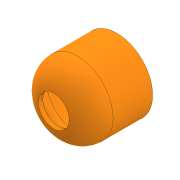
# Autodesk Inventor part: Axis 6 Gearbox
Saved by Autodesk Inventor 2020 (Build 240168000, 168)
## iProperties
Created: 2021-06-29
Part Number: Axis 6 Gearbox
Material: Generic
Document SubType Name: Modeling
Designer: Coy
Density: 1 g/cm^3
Appearance: Orange
Author: Coy
Autodesk Inventor part; units mm, degrees
ref_plane "YZ Plane" through (0, 0, 0) normal (1, 0, 0) x (0, 1, 0)
ref_plane "XZ Plane" through (0, 0, 0) normal (0, 1, 0) x (-1, 0, 0)
ref_plane "XY Plane" through (0, 0, 0) normal (0, 0, 1) x (1, 0, 0)
sketch "Sketch1" plane through (0, 0, 0) normal (0, 0, 1) x (1, 0, 0)
  circle A0 centre (0, 0) radius 6
  dimension "d0" = 12
  constraints: 1 centre point, 1 coincident
  measures "d0" diameter of A0
extrude "Extrusion1" add sketch "Sketch1" against normal blind 8
chamfer "Chamfer1" distance 8 angle 2 1 edges at (-6, 0, -8) measured on face at (-6, 0, -7.5)
sketch "Sketch2" plane through (0, 0, -8) normal (0, 0, -1) x (-1, 0, 0)
  circle A0 centre (0, 0) radius 6 construction
  circle A1 centre (0, 0) radius 5.7206 projected
  line L0 (0, 0) -> (0, 8.298) construction
  arc A2 (0.1999, 5.9933) -> (-0.1999, 5.9933) centre (0, 6) ccw
  line L1 (0.1907, 5.7175) -> (0.2, 5.9967)
  line L2 (-0.1907, 5.7175) -> (-0.2, 5.9967)
  arc A3 (-5.0904, 3.1698) -> (-5.2903, 2.8236) centre (-5.1962, 3) ccw
  line L3 (-5.0468, 2.6936) -> (-5.2933, 2.8251)
  line L4 (-4.8561, 3.0239) -> (-5.0933, 3.1715)
  arc A4 (-5.2903, -2.8236) -> (-5.0904, -3.1698) centre (-5.1962, -3) ccw
  line L5 (-4.8561, -3.0239) -> (-5.0933, -3.1715)
  line L6 (-5.0468, -2.6936) -> (-5.2933, -2.8251)
  arc A5 (-0.1999, -5.9933) -> (0.1999, -5.9933) centre (0, -6) ccw
  line L7 (0.1907, -5.7175) -> (0.2, -5.9967)
  line L8 (-0.1907, -5.7175) -> (-0.2, -5.9967)
  arc A6 (5.0904, -3.1698) -> (5.2903, -2.8236) centre (5.1962, -3) ccw
  line L9 (5.0468, -2.6936) -> (5.2933, -2.8251)
  line L10 (4.8561, -3.0239) -> (5.0933, -3.1715)
  arc A7 (5.2903, 2.8236) -> (5.0904, 3.1698) centre (5.1962, 3) ccw
  line L11 (4.8561, 3.0239) -> (5.0933, 3.1715)
  line L12 (5.0468, 2.6936) -> (5.2933, 2.8251)
  dimension "d6" = 0.4
  dimension "d9" = 360
  constraints: 26 end point, 17 point on circle, 13 point on line, 6 centre point, 2 line through centre, 2 tangent, 1 vertical, 61 other
  measures "d6" diameter of A2
extrude "Extrusion2" add sketch "Sketch2" against normal up to surface (8 mm away) contours A1 L11 A7 L12 | L9 A6 L10 A1 | A1 L2 A2 L1 | L7 A5 L8 A1 | A1 L3 A3 L4 | L5 A4 L6 A1
sketch "Sketch3" plane through (0, 0, 0) normal (0, 0, 1) x (1, 0, 0)
  arc A0 (-0.2, 5.9967) -> (-5.0933, 3.1715) centre (0, 0) ccw projected
  arc A1 (-5.0933, 3.1715) -> (-5.2933, 2.8252) centre (-5.1962, 3) ccw projected
  arc A2 (-5.2933, 2.8252) -> (-5.2933, -2.8252) centre (0, 0) ccw projected
  arc A3 (-5.2933, -2.8252) -> (-5.0933, -3.1715) centre (-5.1962, -3) ccw projected
  arc A4 (-5.0933, -3.1715) -> (-0.2, -5.9967) centre (0, 0) ccw projected
  arc A5 (-0.2, -5.9967) -> (0.2, -5.9967) centre (0, -6) ccw projected
  arc A6 (0.2, -5.9967) -> (5.0933, -3.1715) centre (0, 0) ccw projected
  arc A7 (5.0933, -3.1715) -> (5.2933, -2.8252) centre (5.1962, -3) ccw projected
  arc A8 (5.2933, -2.8252) -> (5.2933, 2.8252) centre (0, 0) ccw projected
  arc A9 (5.2933, 2.8252) -> (5.0933, 3.1715) centre (5.1962, 3) ccw projected
  arc A10 (5.0933, 3.1715) -> (0.2, 5.9967) centre (0, 0) ccw projected
  arc A11 (0.2, 5.9967) -> (-0.2, 5.9967) centre (0, 6) ccw projected
extrude "Extrusion3" add sketch "Sketch3" along normal blind 0.5
sketch "Sketch4" plane through (0, 0, 0.5) normal (0, 0, 1) x (1, 0, 0)
  circle A0 centre (0, 0) radius 32.5
  dimension "d15" = 65
  constraints: 1 centre point, 1 coincident
  measures "d15" diameter of A0
extrude "Extrusion4" add sketch "Sketch4" along normal blind 4
sketch "Sketch5" plane through (0, 0, 4.5) normal (0, 0, 1) x (1, 0, 0)
  circle A0 centre (0, 0) radius 32.5
  circle A1 centre (0, 0) radius 28.5
  dimension "d18" = 4
  constraints: 2 centre point, 1 coincident
  measures "d18" radial gap between concentric circles of A0 A1
extrude "Extrusion5" add sketch "Sketch5" along normal blind 32
sketch "Sketch6" plane through (0, 0, 0) normal (1, 0, 0) x (0, 1, 0)
  line L0 (2.6936, -8) -> (-2.6936, -8) construction
  line L1 (0, -8) -> (0, 93.9815)
  line L2 (-14, 58) -> (14, 58)
  line L3 (32.5, 36.5) -> (-32.5, 36.5) projected
  line L4 (32.5, 0.5) -> (32.5, 36.5) construction
  line L5 (-32.5, 0.5) -> (-32.5, 36.5) construction
  arc A0 (32.5, 36.5) -> (14, 58) centre (10.7568, 36.5) ccw
  arc A1 (28.5, 36.5) -> (13.6847, 54) centre (10.7568, 36.5) ccw
  line L6 (13.6847, 54) -> (-14, 54)
  line L7 (14, 58) -> (14, 40.3088)
  point P0 (0, 0)
  point P1 (0, 58)
  point P2 (0, 54)
  point P3 (14, 53.9443)
  dimension "d21" = 28
  dimension "d22" = 14
  dimension "d23" = 21.5
  dimension "d24" = 4
  constraints: 8 end point, 4 point on circle, 3 vertical, 2 centre point, 1 horizontal, 1 midpoint, 1 tangent, 1 other
  measures "d21" distance of L2.start L2.end
  measures "d22" distance from line of L1 L2.end
  measures "d23" distance between parallel lines of L3 L2
  measures "d24" radial gap between concentric circles of A0 A1
revolve "Revolution1" add sketch "Sketch6" angle 360 about axis through (0, 0, -8) along (0, 0, 1) contours A1 L7 A0 L3
equation "\"d22\" = 0.5 * d21"
body "Solid1"
